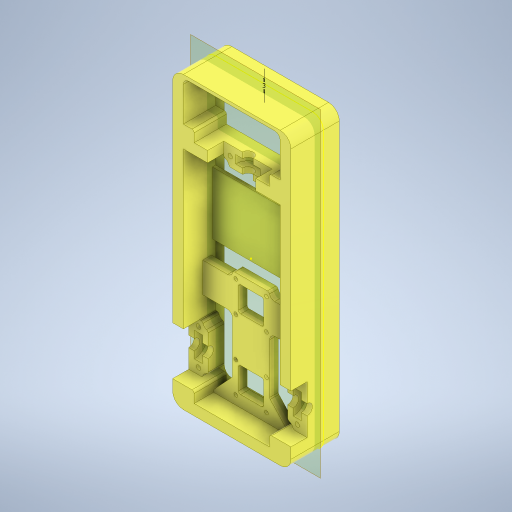
# Autodesk Inventor part: bottom_chassis_extended_v2
Saved by Autodesk Inventor 2024 (Build 280153000, 153)
## iProperties
Created: 2023-09-04
Part Number: bottom_chassis_extended_v2
Material: Generic
Document SubType Name: Modeling
Designer: Pintu
Density: 1 g/cm^3
Appearance: Smooth - Yellow
Author: Pintu
Autodesk Inventor part; units mm, degrees
ref_plane "YZ Plane" through (0, 0, 0) normal (1, 0, 0) x (0, 1, 0)
ref_plane "XZ Plane" through (0, 0, 0) normal (0, 1, 0) x (-1, 0, 0)
ref_plane "XY Plane" through (0, 0, 0) normal (0, 0, 1) x (1, 0, 0)
sketch "Sketch1" plane through (0, 0, 0) normal (0, 0, 1) x (1, 0, 0)
  line L0 (-55, 135) -> (55, 135)
  line L1 (55, 135) -> (55, -135)
  line L2 (55, -135) -> (-55, -135)
  line L3 (-55, -135) -> (-55, 135)
  line L4 (-55, 135) -> (55, -135) construction
  line L5 (55, 135) -> (-55, -135) construction
  line L6 (-45, -125) -> (-45, 132)
  line L7 (-45, 132) -> (45, 132)
  line L8 (45, 132) -> (45, -125)
  line L9 (45, -125) -> (-45, -125)
  line L10 (-55, 135) -> (-37, 135)
  line L11 (-37, 135) -> (-37, 117)
  line L12 (-37, 117) -> (-55, 117)
  line L13 (-55, 117) -> (-55, 135)
  line L14 (-55, -135) -> (-37, -135)
  line L15 (-37, -135) -> (-37, -117)
  line L16 (-37, -117) -> (-55, -117)
  line L17 (-55, -117) -> (-55, -135)
  line L18 (55, -135) -> (37, -135)
  line L19 (37, -135) -> (37, -117)
  line L20 (37, -117) -> (55, -117)
  line L21 (55, -117) -> (55, -135)
  line L22 (55, 135) -> (37, 135)
  line L23 (37, 135) -> (37, 117)
  line L24 (37, 117) -> (55, 117)
  line L25 (55, 117) -> (55, 135)
  point P0 (0, 0)
  point P1 (-37, -125)
  point P2 (-45, -117)
  point P3 (-45, 117)
  point P4 (-37, 132)
  point P5 (37, 132)
  point P6 (45, 117)
  point P7 (45, -117)
  point P8 (37, -125)
  dimension "d0" = 110
  dimension "d1" = 270
  dimension "d2" = 10
  dimension "d3" = 10
  dimension "d4" = 10
  dimension "d5" = 3
  dimension "shaft" = 18
  dimension "d7" = 18
  dimension "d8" = 18
  dimension "d9" = 18
  dimension "d10" = 18
  dimension "d11" = 18
  dimension "d12" = 18
  dimension "d13" = 18
  constraints: 52 end point, 12 parallel, 6 perpendicular, 5 horizontal, 2 midpoint, 1 vertical
  measures "d0" distance of L1.end L2.end
  measures "d1" distance of L0.end L1.end
  measures "d2" distance between parallel lines of L1 L8
  measures "d3" distance between parallel lines of L3 L6
  measures "d4" distance between parallel lines of L2 L9
  measures "d5" distance between parallel lines of L0 L7
  measures "shaft" distance of L11.end L12.end
  measures "d7" distance of L10.end L11.end
  measures "d8" distance of L16.end L15.end
  measures "d9" distance of L15.end L14.end
  measures "d10" distance of L19.end L20.end
  measures "d11" distance of L18.end L19.end
  measures "d12" distance of L24.end L23.end
  measures "d13" distance of L23.end L22.end
extrude "Extrusion1" add sketch "Sketch1" along normal blind 30 contours L0 L11 L7 L6 L12 L3 | L0 L23 L7 L11 | L12 L6 L16 L3 | L0 L1 L24 L8 L7 L23 | L16 L6 L9 L15 L2 L3 | L16 L15 L9 L6 | L1 L20 L8 L24 | L15 L9 L19 L2 | L1 L2 L19 L9 L8 L20 | L8 L9 L19 L20
sketch "Sketch2" plane through (0, 0, 30) normal (0, 0, 1) x (1, 0, 0)
  line L0 (-55, 135) -> (-55, -135) projected
  line L1 (-55, -70) -> (-37, -70)
  line L2 (-37, -70) -> (-37, -115)
  line L3 (-37, -115) -> (-55, -115)
  line L4 (-55, -115) -> (-55, -70)
  line L5 (-55, -135) -> (55, -135) projected
  line L6 (55, -135) -> (55, 135) projected
  line L7 (55, -115) -> (37, -115)
  line L8 (37, -115) -> (37, -70)
  line L9 (37, -70) -> (55, -70)
  line L10 (55, -70) -> (55, -115)
  point P0 (0, 0)
  dimension "wheelHolderBreath" = 18
  dimension "wheelHolderlength" = 45
  dimension "DistanceWH" = 20
  dimension "d19" = 18
  dimension "d20" = 45
  dimension "d21" = 20
  constraints: 16 end point, 4 parallel, 2 horizontal, 2 perpendicular, 2 point on line
  measures "wheelHolderBreath" distance of L2.end L3.end
  measures "wheelHolderlength" distance of L1.end L2.end
  measures "DistanceWH" distance between parallel lines of L5 L3
  measures "d19" distance of L8.end L9.end
  measures "d20" distance of L7.end L8.end
  measures "d21" distance between parallel lines of L5 L7
extrude "Extrusion2" add sketch "Sketch2" against normal blind 30
fillet "Fillet1" radius 5 4 edges at (-37, -70, 15) (-37, -115, 15) (37, -70, 15) (37, -115, 15) inverted yes
fillet "Fillet2" radius 2 8 edges at (-42, -70, 15) (-42, -115, 15) (42, -115, 15) (42, -70, 15) (-37, -75, 15) (-37, -110, 15) (37, -110, 15) (37, -75, 15)
extrude "Extrusion3" cut sketch "Sketch2" against normal blind 15
ref_plane "Work Plane1" through (-46, -108.2918, 0) normal (1, 0, 0) x (0, 0, -1)
sketch "Sketch3" plane through (-46, -108.2918, 0) normal (1, 0, 0) x (0, 0, -1)
  line L0 (-30, -6.7082) -> (-15, -6.7082) projected
  line L1 (-15, -6.7082) -> (-15, 38.2918) projected
  line L2 (-15, 38.2918) -> (-30, 38.2918) projected
  line L3 (-30, 243.2918) -> (-30, 38.2918) projected
  line L4 (0, 243.2918) -> (-30, 243.2918) projected
  line L5 (0, 243.2918) -> (0, -26.7082) projected
  line L6 (0, -26.7082) -> (-30, -26.7082) projected
  line L7 (-30, -6.7082) -> (-30, -26.7082) projected
  line L8 (-15, 38.2918) -> (-30, 38.2918) projected
  line L9 (-30, -6.7082) -> (-15, -6.7082) projected
  line L10 (-15, -6.7082) -> (-15, 38.2918) projected
  circle A0 centre (-15, 15.7918) radius 11.5
  point P0 (0, 108.2918)
  dimension "d28" = 23
  constraints: 1 centre point, 1 midpoint
  measures "d28" diameter of A0
extrude "Extrusion4" cut sketch "Sketch3" along normal mid plane 7.5 contours A0 L1 | L1 A0
ref_plane "Work Plane2" through (-39.625, -108.2918, 0) normal (1, 0, 0) x (0, 0, -1)
sketch "Sketch4" plane through (-39.625, -108.2918, 0) normal (1, 0, 0) x (0, 0, -1)
  line L0 (-15, 27.2918) -> (-15, 4.2918) projected
  line L1 (-15, 27.2918) -> (-15, 4.2918) projected
  arc A0 (-15, 4.2918) -> (-15, 27.2918) centre (-15, 15.7918) ccw projected
  circle A1 centre (-15, 15.7918) radius 5
  point P0 (0, 108.2918)
  dimension "d31" = 10
  constraints: 1 centre point, 1 coincident
  measures "d31" diameter of A1
extrude "Extrusion5" cut sketch "Sketch4" along normal mid plane 50 contours A1 L0 | L0 A1
ref_plane "Work Plane3" through (0, -135, 0) normal (1, 0, 0) x (0, 0, -1)
mirror "Mirror1" about plane through (0, -135, 0) normal (1, 0, 0) of "Extrusion3", "Extrusion5", "Extrusion4"
sketch "Sketch7" plane through (0, 0, 0) normal (0, 0, -1) x (-1, 0, 0)
  arc A0 (-37, -76.7082) -> (-38.4286, -74.7916) centre (-39, -76.7082) ccw projected
  arc A1 (-41.7916, -71.4286) -> (-38.4286, -74.7916) centre (-37, -70) ccw projected
  arc A2 (-41.7916, -71.4286) -> (-43.7082, -70) centre (-43.7082, -72) ccw projected
  line L0 (-43.7082, -70) -> (-45, -70) projected
  line L1 (-45, 132) -> (-45, -70) projected
  line L2 (45, 132) -> (-45, 132) projected
  line L3 (45, -70) -> (45, 132) projected
  line L4 (45, -70) -> (43.7082, -70) projected
  arc A3 (43.7082, -70) -> (41.7916, -71.4286) centre (43.7082, -72) ccw projected
  arc A4 (38.4286, -74.7916) -> (41.7916, -71.4286) centre (37, -70) ccw projected
  arc A5 (38.4286, -74.7916) -> (37, -76.7082) centre (39, -76.7082) ccw projected
  line L5 (37, -76.7082) -> (37, -108.2918) projected
  arc A6 (37, -108.2918) -> (38.4286, -110.2084) centre (39, -108.2918) ccw projected
  arc A7 (41.7916, -113.5714) -> (38.4286, -110.2084) centre (37, -115) ccw projected
  arc A8 (41.7916, -113.5714) -> (43.7082, -115) centre (43.7082, -113) ccw projected
  line L6 (43.7082, -115) -> (45, -115) projected
  line L7 (45, -117) -> (45, -115) projected
  line L8 (37, -117) -> (45, -117) projected
  line L9 (37, -125) -> (37, -117) projected
  line L10 (-37, -125) -> (37, -125) projected
  line L11 (-37, -117) -> (-37, -125) projected
  line L12 (-45, -117) -> (-37, -117) projected
  line L13 (-45, -115) -> (-45, -117) projected
  line L14 (-45, -115) -> (-43.7082, -115) projected
  arc A9 (-43.7082, -115) -> (-41.7916, -113.5714) centre (-43.7082, -113) ccw projected
  arc A10 (-38.4286, -110.2084) -> (-41.7916, -113.5714) centre (-37, -115) ccw projected
  arc A11 (-38.4286, -110.2084) -> (-37, -108.2918) centre (-39, -108.2918) ccw projected
  line L15 (-37, -108.2918) -> (-37, -76.7082) projected
  line L16 (-55, -135) -> (-55, 135) projected
  line L17 (55, -135) -> (-55, -135) projected
  line L18 (55, 135) -> (55, -135) projected
  line L19 (-55, 135) -> (55, 135) projected
  line L20 (-55, 85) -> (55, 85)
  line L21 (55, 85) -> (55, 75)
  line L22 (55, 75) -> (-55, 75)
  line L23 (-55, 75) -> (-55, 85)
  point P0 (0, 0)
  point P1 (-55, 75)
  dimension "d54" = 10
  dimension "d55" = 220
  constraints: 8 end point, 2 parallel, 2 perpendicular, 2 point on line
  measures "d54" distance of L20.end L21.end
  measures "d55" distance between parallel lines of L17 L20
extrude "Extrusion7" add sketch "Sketch7" against normal blind 30 contours L22 L16 L20 L1 | L1 L20 L3 L22 | L3 L20 L18 L22
sketch "Sketch8" plane through (0, 0, 30) normal (0, 0, 1) x (1, 0, 0)
  line L0 (45, 75) -> (45, -70) projected
  line L1 (45, -70) -> (55, -70) projected
  line L2 (55, -70) -> (55, 135) projected
  line L3 (55, 135) -> (-55, 135) projected
  line L4 (-55, 135) -> (-55, -70) projected
  line L5 (-55, -70) -> (-45, -70) projected
  line L6 (-45, -70) -> (-45, 75) projected
  line L7 (-45, 75) -> (45, 75) projected
  line L8 (45, 85) -> (-45, 85) projected
  line L9 (-45, 85) -> (-45, 132) projected
  line L10 (-45, 132) -> (45, 132) projected
  line L11 (45, 132) -> (45, 85) projected
  line L12 (-22.5, 85) -> (22.5, 85)
  line L13 (22.5, 85) -> (22.5, 67)
  line L14 (22.5, 67) -> (-22.5, 67)
  line L15 (-22.5, 67) -> (-22.5, 85)
  line L16 (0, 85) -> (0, 75) construction
  line L17 (55, -115) -> (45, -115) projected
  line L18 (45, -115) -> (45, -117) projected
  line L19 (45, -117) -> (37, -117) projected
  line L20 (37, -117) -> (37, -125) projected
  line L21 (37, -125) -> (-37, -125) projected
  line L22 (-37, -125) -> (-37, -117) projected
  line L23 (-37, -117) -> (-45, -117) projected
  line L24 (-45, -117) -> (-45, -115) projected
  line L25 (-45, -115) -> (-55, -115) projected
  line L26 (-55, -115) -> (-55, -135) projected
  line L27 (-55, -135) -> (55, -135) projected
  line L28 (55, -135) -> (55, -115) projected
  point P0 (0, 0)
  point P1 (0, 80)
  dimension "d58" = 18
  dimension "d59" = 45
  dimension "d60" = 22.5
  constraints: 10 end point, 3 midpoint, 2 parallel, 2 point on line, 1 perpendicular
  measures "d58" distance of L12.end L13.end
  measures "d59" distance between parallel lines of L13 L15
  measures "d60" distance from line of point (0, 80) L13
extrude "Extrusion8" add sketch "Sketch8" against normal blind 30 contours L13 L14 L15 L7 | L7 L15 L8 L13
extrude "Extrusion9" cut sketch "Sketch8" against normal blind 15 contours L13 L14 L15 L7 | L7 L15 L8 L13
sketch "Sketch10" plane through (0, 0, 0) normal (0, 0, -1) x (-1, 0, 0)
  line L0 (55, 135) -> (55, -135) projected
  line L1 (45, -70) -> (43.7082, -70) projected
  point P0 (0, 0)
  point P1 (46, -76)
  dimension "d66" = 9
  dimension "d67" = 6
  measures "d66" distance from line of L0 point (46, -76)
  measures "d67" distance from line of L1 point (46, -76)
hole "Hole3" at (-46, -76, 0) direction (0, 0, 1) diameter 4.2 end through all
sketch "Sketch11" plane through (0, 0, 0) normal (0, 0, -1) x (-1, 0, 0)
  line L0 (55, 135) -> (55, -135) projected
  line L1 (43.7082, -115) -> (45, -115) projected
  point P0 (0, 0)
  point P1 (46, -109)
  dimension "d75" = 9
  dimension "d76" = 6
  measures "d75" distance from line of L0 point (46, -109)
  measures "d76" distance from line of L1 point (46, -109)
hole "Hole4" at (-46, -109, 0) direction (0, 0, 1) diameter 4.2 end through all
sketch "Sketch12" plane through (0, 0, 0) normal (0, 0, -1) x (-1, 0, 0)
  circle A0 centre (46, -76) radius 2.1 projected
  circle A1 centre (46, -109) radius 2.1 projected
  line L0 (49.5218, -78.0333) -> (46, -80.0667)
  line L1 (46, -80.0667) -> (42.4782, -78.0333)
  line L2 (42.4782, -78.0333) -> (42.4782, -73.9667)
  line L3 (42.4782, -73.9667) -> (46, -71.9333)
  line L4 (46, -71.9333) -> (49.5218, -73.9667)
  line L5 (49.5218, -73.9667) -> (49.5218, -78.0333)
  line L6 (49.5218, -111.0333) -> (46, -113.0667)
  line L7 (46, -113.0667) -> (42.4782, -111.0333)
  line L8 (42.4782, -111.0333) -> (42.4782, -106.9667)
  line L9 (42.4782, -106.9667) -> (46, -104.9333)
  line L10 (46, -104.9333) -> (49.5218, -106.9667)
  line L11 (49.5218, -106.9667) -> (49.5218, -111.0333)
  line L12 (37, -76.7082) -> (37, -108.2918) projected
  point P0 (0, 0)
  point P1 (44.2391, -79.05)
  point P2 (47.7609, -72.95)
  point P3 (44.2391, -112.05)
  point P4 (47.7609, -105.95)
  point P5 (47.7609, -79.05)
  point P6 (47.7609, -112.05)
  dimension "d136" = 3.05
  dimension "d137" = 3.05
  constraints: 24 end point, 6 midpoint, 2 coincident, 2 parallel, 26 other
  measures "d136" vertical distance of point (47.761, -79.05) A0.centre
  measures "d137" vertical distance of point (47.761, -112.05) A1.centre
extrude "Extrusion10" cut sketch "Sketch12" against normal blind 3 contours A0 | A1 | L0 L1 L2 L3 L4 L5 | L6 L7 L8 L9 L10 L11
mirror "Mirror2" about plane through (0, -135, 0) normal (1, 0, 0) of "Extrusion10", "Hole3", "Hole4"
ref_plane "Work Plane5" through (-22.5, 76, 0) normal (0, -1, 0) x (1, 0, 0)
sketch "Sketch13" plane through (-22.5, 76, 0) normal (0, -1, 0) x (1, 0, 0)
  line L0 (45, 15) -> (0, 15) projected
  line L1 (0, 15) -> (0, 0) projected
  line L2 (45, 0) -> (0, 0) projected
  line L3 (45, 15) -> (45, 0) projected
  circle A0 centre (22.5, 15) radius 11.5
  point P0 (22.5, 0)
  dimension "bearing" = 23
  constraints: 1 centre point, 1 midpoint
  measures "bearing" diameter of A0
extrude "Extrusion11" cut sketch "Sketch13" along normal mid plane 7.5 contours A0 L0 | L0 A0
sketch "Sketch14" plane through (-22.5, 76, 0) normal (0, -1, 0) x (1, 0, 0)
  line L0 (34, 15) -> (11, 15) projected
  arc A0 (11, 15) -> (34, 15) centre (22.5, 15) ccw projected
  circle A1 centre (22.5, 15) radius 5
  point P0 (22.5, 0)
  dimension "d91" = 10
  constraints: 1 centre point, 1 coincident
  measures "d91" diameter of A1
extrude "Extrusion12" cut sketch "Sketch14" along normal mid plane 50 contours A1 L0 | L0 A1
fillet "Fillet3" radius 5 2 edges at (22.5, 67, 7.5) (-22.5, 67, 7.5) inverted yes
fillet "Fillet4" radius 2 4 edges at (17.5, 67, 7.5) (22.5, 72, 7.5) (-17.5, 67, 7.5) (-22.5, 72, 7.5)
sketch "Sketch17" plane through (0, 0, 0) normal (0, 0, -1) x (-1, 0, 0)
  line L0 (22.5, 73.7082) -> (22.5, 75) projected
  line L1 (-15.7918, 67) -> (15.7918, 67) projected
  point P0 (0, 0)
  point P1 (16.5, 76)
  dimension "d114" = 6
  dimension "d115" = 9
  measures "d114" distance from line of L0 point (16.5, 76)
  measures "d115" distance from line of L1 point (16.5, 76)
hole "Hole7" at (-16.5, 76, 0) direction (0, 0, 1) diameter 4.2 end through all
sketch "Sketch18" plane through (0, 0, 0) normal (0, 0, -1) x (-1, 0, 0)
  line L0 (-15.7918, 67) -> (15.7918, 67) projected
  line L1 (-22.5, 75) -> (-22.5, 73.7082) projected
  point P0 (0, 0)
  point P1 (-16.5, 76)
  dimension "d123" = 9
  dimension "d124" = 6
  measures "d123" distance from line of L0 point (-16.5, 76)
  measures "d124" distance from line of L1 point (-16.5, 76)
hole "Hole8" at (16.5, 76, 0) direction (0, 0, 1) diameter 4.2 end through all
sketch "Sketch19" plane through (0, 0, 0) normal (0, 0, -1) x (-1, 0, 0)
  circle A0 centre (16.5, 76) radius 2.1 projected
  circle A1 centre (-16.5, 76) radius 2.1 projected
  line L0 (14.7391, 79.05) -> (18.2609, 79.05)
  line L1 (18.2609, 79.05) -> (20.0218, 76)
  line L2 (20.0218, 76) -> (18.2609, 72.95)
  line L3 (18.2609, 72.95) -> (14.7391, 72.95)
  line L4 (14.7391, 72.95) -> (12.9782, 76)
  line L5 (12.9782, 76) -> (14.7391, 79.05)
  line L6 (-18.2609, 79.05) -> (-14.7391, 79.05)
  line L7 (-14.7391, 79.05) -> (-12.9782, 76)
  line L8 (-12.9782, 76) -> (-14.7391, 72.95)
  line L9 (-14.7391, 72.95) -> (-18.2609, 72.95)
  line L10 (-18.2609, 72.95) -> (-20.0218, 76)
  line L11 (-20.0218, 76) -> (-18.2609, 79.05)
  line L12 (-15.7918, 67) -> (15.7918, 67) projected
  point P0 (0, 0)
  point P1 (16.5, 79.05)
  point P2 (-16.5, 79.05)
  dimension "d132" = 3.05
  dimension "d133" = 3.05
  constraints: 24 end point, 2 coincident, 2 midpoint, 2 parallel, 26 other
  measures "d132" distance of point (16.5, 79.05) A0.centre
  measures "d133" distance of point (-16.5, 79.05) A1.centre
extrude "Extrusion13" cut sketch "Sketch19" against normal blind 3 contours A0 | L0 L1 L2 L3 L4 L5 | L6 L7 L8 L9 L10 L11
fillet "Fillet5" radius 10 4 edges at (-55, 135, 15) (55, 135, 15) (-55, -135, 15) (55, -135, 15)
fillet "Fillet6" radius 2 2 edges at (37, -117, 15) (-37, -117, 15)
sketch "Sketch26" plane through (0, 0, 0) normal (0, 0, -1) x (-1, 0, 0)
  line L0 (-45, 132) -> (-45, 85) projected
  line L1 (-55, 75) -> (-35, 75)
  line L2 (-35, 75) -> (-35, 95)
  line L3 (-35, 95) -> (-55, 95)
  line L4 (-55, 95) -> (-55, 75)
  line L5 (-55, 75) -> (-35, 95) construction
  line L6 (-35, 75) -> (-55, 95) construction
  line L7 (55, 75) -> (35, 75)
  line L8 (35, 75) -> (35, 95)
  line L9 (35, 95) -> (55, 95)
  line L10 (55, 95) -> (55, 75)
  line L11 (45, 85) -> (45, 132) projected
  line L12 (55, 75) -> (35, 95) construction
  line L13 (35, 75) -> (55, 95) construction
  point P0 (0, 0)
  point P1 (-45, 117)
  point P2 (45, 117)
  dimension "d188" = 20
  dimension "d189" = 20
  dimension "d190" = 20
  dimension "d191" = 20
  constraints: 24 end point, 4 midpoint, 4 parallel, 2 horizontal, 2 perpendicular
  measures "d188" distance of L3.end L2.end
  measures "d189" distance of L2.end L1.end
  measures "d190" distance of L8.end L9.end
  measures "d191" distance of L7.end L8.end
extrude "Extrusion16" add sketch "Sketch26" against normal blind 30
fillet "Fillet7" radius 2 2 edges at (35, 95, 15) (-35, 95, 15)
sketch "Sketch27" plane through (0, 0, 0) normal (0, 0, -1) x (-1, 0, 0)
  line L0 (-45, 132) -> (-45, 95) projected
  circle A0 centre (-45, 85) radius 5
  line L1 (-45, 75) -> (-22.5, 75) projected
  line L2 (-35, 85) -> (-35, 93) projected
  circle A1 centre (-45, -125) radius 5
  line L3 (45, -135) -> (-45, -135) projected
  line L4 (-55, -125) -> (-55, 125) projected
  line L5 (-45, 135) -> (45, 135) construction
  line L6 (0, 135) -> (0, -135) construction
  circle A2 centre (45, 85) radius 5
  circle A3 centre (45, -125) radius 5
  point P0 (0, 0)
  point P1 (-45, 117)
  dimension "shaftODcut" = 10
  dimension "shaftCutDist" = 10
  dimension "d197" = 10
  dimension "d199" = 10
  dimension "d200" = 10
  dimension "d201" = 10
  constraints: 4 centre point, 2 end point, 2 midpoint, 2 symmetric about line, 2 other
  measures "shaftODcut" diameter of A0
  measures "shaftCutDist" distance from line of L1 A0.centre
  measures "d197" distance from line of L2 A0.centre
  measures "d199" diameter of A1
  measures "d200" distance from line of L3 A1.centre
  measures "d201" distance from line of L4 A1.centre
fillet "Fillet8" radius 5 2 edges at (45, 132, 15) (-45, 132, 15)
extrude "Extrusion17" cut sketch "Sketch27" against normal blind 25
ref_plane "Work Plane7" through (0, 0, 8) normal (0, 0, -1) x (-1, 0, 0)
sketch "Sketch30" plane through (0, 0, 8) normal (0, 0, -1) x (-1, 0, 0)
  line L0 (-37, -125) -> (37, -125) projected
  arc A0 (39, -117) -> (37, -119) centre (39, -119) ccw projected
  line L1 (39, -117) -> (45, -117) projected
  line L2 (45, -117) -> (45, -115) projected
  line L3 (45, -115) -> (55, -115) projected
  line L4 (55, -115) -> (55, -125) projected
  arc A1 (45, -135) -> (55, -125) centre (45, -125) ccw projected
  line L5 (45, -135) -> (-45, -135) projected
  arc A2 (-55, -125) -> (-45, -135) centre (-45, -125) ccw projected
  line L6 (-55, -125) -> (-55, -115) projected
  line L7 (-55, -115) -> (-45, -115) projected
  line L8 (-45, -115) -> (-45, -117) projected
  line L9 (-45, -117) -> (-39, -117) projected
  arc A3 (-37, -119) -> (-39, -117) centre (-39, -119) ccw projected
  line L10 (-37, -119) -> (-37, -125) projected
  line L11 (-37, -125) -> (37, -125) projected
  line L12 (37, -125) -> (37, -119) projected
  line L13 (0, -135) -> (0, -12.5) construction
  line L14 (17.25, -20.25) -> (-17.25, -20.25)
  line L15 (-17.25, -20.25) -> (-17.25, -54.75)
  line L16 (-17.25, -54.75) -> (17.25, -54.75)
  line L17 (17.25, -54.75) -> (17.25, -20.25)
  line L18 (17.25, -20.25) -> (-17.25, -54.75) construction
  line L19 (-17.25, -20.25) -> (17.25, -54.75) construction
  line L20 (17.25, -85.25) -> (-17.25, -85.25)
  line L21 (-17.25, -85.25) -> (-17.25, -119.75)
  line L22 (-17.25, -119.75) -> (17.25, -119.75)
  line L23 (17.25, -119.75) -> (17.25, -85.25)
  line L24 (17.25, -85.25) -> (-17.25, -119.75) construction
  line L25 (-17.25, -85.25) -> (17.25, -119.75) construction
  circle A4 centre (14.25, -23.25) radius 1.75
  line L26 (17.25, -37.5) -> (-17.25, -37.5) construction
  line L27 (17.25, -102.5) -> (-17.25, -102.5) construction
  circle A5 centre (-14.25, -23.25) radius 1.75
  circle A6 centre (14.25, -51.75) radius 1.75
  circle A7 centre (-14.25, -51.75) radius 1.75
  circle A8 centre (14.25, -88.25) radius 1.75
  circle A9 centre (-14.25, -88.25) radius 1.75
  circle A10 centre (14.25, -116.75) radius 1.75
  circle A11 centre (-14.25, -116.75) radius 1.75
  line L28 (45, -23.5) -> (-45, -23.5)
  line L29 (-45, -23.5) -> (-45, -51.5)
  line L30 (-45, -51.5) -> (45, -51.5)
  line L31 (45, -51.5) -> (45, -23.5)
  line L32 (45, -23.5) -> (-45, -51.5) construction
  line L33 (-45, -23.5) -> (45, -51.5) construction
  line L34 (17.25, -54.75) -> (-17.25, -54.75)
  line L35 (-17.25, -54.75) -> (-17.25, -125)
  line L36 (-17.25, -125) -> (17.25, -125)
  line L37 (17.25, -125) -> (17.25, -54.75)
  line L38 (11.75, -25.75) -> (-11.75, -25.75)
  line L39 (-11.75, -25.75) -> (-11.75, -49.25)
  line L40 (-11.75, -49.25) -> (11.75, -49.25)
  line L41 (11.75, -49.25) -> (11.75, -25.75)
  line L42 (11.75, -90.75) -> (-11.75, -90.75)
  line L43 (-11.75, -90.75) -> (-11.75, -114.25)
  line L44 (-11.75, -114.25) -> (11.75, -114.25)
  line L45 (11.75, -114.25) -> (11.75, -90.75)
  line L46 (0, -85.25) -> (37, -125)
  line L47 (-37, -125) -> (0, -85.25)
  point P0 (0, 0)
  point P1 (0, -37.5)
  point P2 (0, -102.5)
  point P3 (17.25, -51.5)
  point P4 (17.25, -23.5)
  point P5 (-17.25, -23.5)
  point P6 (-17.25, -51.5)
  point P7 (-18, -55.5)
  point P8 (-17.25, -85.25)
  point P9 (-17.25, -103.7821)
  point P10 (17.25, -103.7821)
  point P11 (17.25, -85.25)
  point P12 (-17.25, -85.25)
  point P13 (17.25, -85.25)
  point P14 (17.25, -119.75)
  point P15 (-17.25, -119.75)
  point P16 (17.25, -103.7821)
  point P17 (-17.25, -103.7821)
  point P18 (-17.25, -125)
  point P19 (17.25, -125)
  point P20 (-17.25, -119.75)
  point P21 (17.25, -119.75)
  point P22 (-5.1195, -90.75)
  point P23 (-11.75, -97.8733)
  point P24 (11.75, -97.8733)
  point P25 (5.1195, -90.75)
  dimension "d223" = 122.5
  dimension "d224" = 34.5
  dimension "d225" = 34.5
  dimension "d226" = 34.5
  dimension "d227" = 34.5
  dimension "d228" = 25
  dimension "d229" = 65
  dimension "d230" = 3.5
  dimension "screwDist" = 3
  dimension "d232" = 3
  dimension "d233" = 3.5
  dimension "d234" = 3
  dimension "d235" = 3
  dimension "d236" = 90
  dimension "d237" = 28
  dimension "d238" = 5.5
  dimension "d239" = 5.5
  constraints: 70 end point, 12 midpoint, 12 parallel, 8 centre point, 6 perpendicular, 6 symmetric about line, 4 horizontal, 3 point on line, 1 vertical, 12 other
  measures "d223" distance of L13.start L13.end
  measures "d224" distance of L16.end L15.end
  measures "d225" distance of L15.end L14.end
  measures "d226" distance of L22.end L21.end
  measures "d227" distance of L21.end L20.end
  measures "d228" distance of point (0, -37.5) L13.end
  measures "d229" distance of point (0, -102.5) point (0, -37.5)
  measures "d230" diameter of A4
  measures "screwDist" distance from line of L14 A4.centre
  measures "d232" distance from line of L17 A4.centre
  measures "d233" diameter of A8
  measures "d234" distance from line of L20 A8.centre
  measures "d235" distance from line of L23 A8.centre
  measures "d236" distance of L30.end L29.end
  measures "d237" distance of L29.end L28.end
  measures "d238" distance between parallel lines of L17 L41
  measures "d239" distance between parallel lines of L23 L45
extrude "Extrusion19" add sketch "Sketch30" along normal mid plane 8 contours L47 L21 L35 L0 | L35 L22 L37 L0 | L47 L43 L44 L45 L46 L23 L22 L21 | L21 L20 L47 L42 L43 | L37 L23 L46 L0 | L35 L16 L37 L20 | L20 L23 L46 L45 L42 | L46 L42 L47 | L15 L30 A7 A6 L17 L16 | L30 L29 L28 L15 | L15 L28 A5 A4 L17 L30 A6 A7 | L15 L14 L17 L28 A4 A5 | L17 L28 L31 L30
fillet "Fillet9" radius 5 4 edges at (-17.25, -51.5, 8) (17.25, -51.5, 8) (-17.25, -23.5, 8) (17.25, -23.5, 8)
move faces "Move1" translate (0, 2, 0) faces at (-5.75, -20.25, 9.3333)
fillet "Fillet10" radius 2 12 edges at (-16.94, -18.25, 8) (16.94, -18.25, 8) (-11.75, -25.75, 8) (11.75, -25.75, 8) (-11.75, -49.25, 8) (11.75, -49.25, 8) (11.75, -90.75, 8) (-11.75, -90.75, 8) (-11.75, -114.25, 8) (11.75, -114.25, 8) (17.25, -103.7821, 8) (-17.25, -103.7821, 8)
sketch "Sketch31" plane through (0, 0, 12) normal (0, 0, 1) x (1, 0, 0)
  point P0 (0, 0)
sketch "Sketch32" plane through (0, 0, 0) normal (0, 0, -1) x (-1, 0, 0)
  line L0 (-45, 75) -> (-45, -70) projected
  line L1 (45, -70) -> (45, 75) projected
  line L2 (-45, 47) -> (45, 47)
  line L3 (45, 47) -> (45, -11)
  line L4 (45, -11) -> (-45, -11)
  line L5 (-45, -11) -> (-45, 47)
  line L6 (-15.7918, 67) -> (15.7918, 67) projected
  point P0 (0, 0)
  point P1 (45, 47)
  dimension "d247" = 58
  dimension "d248" = 20
  constraints: 8 end point, 2 parallel, 2 point on line, 1 horizontal, 1 perpendicular
  measures "d247" distance of L2.end L3.end
  measures "d248" distance between parallel lines of L2 L6
extrude "Extrusion20" add sketch "Sketch32" against normal blind 3
move faces "Move2" translate (0, 2, 0) faces at (-41, -117, 10)
move faces "Move3" translate (2, 0, 0) faces at (-37, -119.6667, 14)
move faces "Move4" translate (0, 2, 0) faces at (43, -117, 10)
move faces "Move5" translate (-2, 0, 0) faces at (37, -119.6667, 14)
sketch "Sketch33" plane through (0, 0, 0) normal (0, 0, -1) x (-1, 0, 0)
  line L0 (-55, -125) -> (-55, 125) projected
  arc A0 (-45, 135) -> (-55, 125) centre (-45, 125) ccw projected
  line L1 (-45, 135) -> (45, 135) projected
  arc A1 (55, 125) -> (45, 135) centre (45, 125) ccw projected
  line L2 (55, 125) -> (55, -125) projected
  arc A2 (45, -135) -> (55, -125) centre (45, -125) ccw projected
  line L3 (45, -135) -> (-45, -135) projected
  arc A3 (-55, -125) -> (-45, -135) centre (-45, -125) ccw projected
  line L4 (45, 132) -> (-45, 132)
  arc A4 (-45, 132) -> (-52, 125) centre (-45, 125) ccw
  line L5 (-52, 125) -> (-52, -125)
  arc A5 (-52, -125) -> (-45, -132) centre (-45, -125) ccw
  line L6 (-45, -132) -> (45, -132)
  arc A6 (45, -132) -> (52, -125) centre (45, -125) ccw
  line L7 (52, -125) -> (52, 125)
  arc A7 (52, 125) -> (45, 132) centre (45, 125) ccw
  point P0 (0, 0)
  dimension "d263" = 3
  constraints: 8 end point, 8 point on circle, 4 centre point, 7 other
  measures "d263" distance between parallel lines of L1 L4
extrude "Extrusion21" add sketch "Sketch33" along normal blind 15 contours L0 A0 L1 A1 L2 A2 L3 A3 | A7 L7 A6 L6 A5 L5 A4 L4
extrude "Extrusion22" cut sketch "Sketch33" along normal blind 15 contours A7 L7 A6 L6 A5 L5 A4 L4
equation "\"d7\" = shaft"
equation "\"d8\" = shaft"
equation "\"d9\" = shaft"
equation "\"d10\" = shaft"
equation "\"d11\" = shaft"
equation "\"d12\" = shaft"
equation "\"d13\" = shaft"
equation "\"d19\" = wheelHolderBreath"
equation "\"d20\" = wheelHolderlength"
equation "\"d21\" = DistanceWH"
equation "\"d58\" = wheelHolderBreath"
equation "\"d59\" = wheelHolderlength"
equation "\"d60\" = 0.5 * wheelHolderlength"
equation "\"d89\" = bearingCut"
equation "\"d197\" = shaftCutDist"
equation "\"bearingCut\" = 7.5"
body "Solid1"
